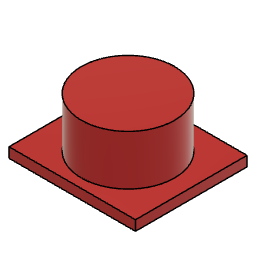
Buttons_V1 (Autodesk Fusion 360 archive; units mm, degrees)
design "ButtonRed"
Autodesk Fusion 360 part; units mm, degrees
(part 1 of 2)
sketch "Sketch1" plane through (0, 45, 0) normal (0, 1, 0) x (-1, 0, 0)
  line L0 (-111.8498, 7.1011) -> (-111.8498, -10.2989)
  line L1 (-111.8498, -10.2989) -> (-134.2498, -10.2989)
  line L2 (-134.2498, -10.2989) -> (-134.2498, 7.1011)
  line L3 (-134.2498, 7.1011) -> (-111.8498, 7.1011)
  circle A0 centre (-138.4498, -1.5989) radius 3.1
  circle A1 centre (-123.0498, 11.3011) radius 3.1
  circle A2 centre (-123.0498, -14.4989) radius 3.1
  circle A3 centre (-107.6498, -1.5989) radius 3.1
  line L4 (-103.4498, -18.6989) -> (-103.4498, 15.5011)
  line L5 (-103.4498, 15.5011) -> (-142.6498, 15.5011)
  line L6 (-142.6498, 15.5011) -> (-142.6498, -18.6989)
  line L7 (-142.6498, -18.6989) -> (-103.4498, -18.6989)
  circle A4 centre (-138.4498, -1.5989) radius 3.1
  circle A5 centre (-123.0498, -14.4989) radius 3.1
  circle A6 centre (-107.6498, -1.5989) radius 3.1
  circle A7 centre (-123.0498, 11.3011) radius 3.1
  line L8 (-154.8498, 7.1011) -> (-154.8498, -10.2989)
  line L9 (-177.2498, -10.2989) -> (-177.2498, 7.1011)
  line L10 (-146.7095, 15.4507) -> (-185.4095, 15.5014)
  line L11 (-177.2498, 7.1011) -> (-154.8498, 7.1011)
  circle A8 centre (-166.0498, -14.4989) radius 3.1
  circle A9 centre (-181.4498, -1.5989) radius 3.1
  line L12 (-185.4095, 15.5014) -> (-185.4536, -18.1986)
  circle A10 centre (-181.4498, -1.5989) radius 3.1
  line L13 (-146.7537, -18.2493) -> (-146.7095, 15.4507)
  circle A11 centre (-166.0498, 11.3011) radius 3.1
  circle A12 centre (-166.0498, 11.3011) radius 3.1
  line L14 (-154.8498, -10.2989) -> (-177.2498, -10.2989)
  circle A13 centre (-150.6498, -1.5989) radius 3.1
  circle A14 centre (-150.6498, -1.5989) radius 3.1
  line L15 (-185.4536, -18.1986) -> (-146.7537, -18.2493)
  circle A15 centre (-166.0498, -14.4989) radius 3.1
  arc A16 (86.5, -27.2432) -> (86.5, -22.3568) centre (88.5, -24.8) ccw
  arc A17 (-86.5, -22.3568) -> (-86.5, -27.2432) centre (-88.5, -24.8) ccw
  line L16 (86.5, 29) -> (-86.5, 29)
  line L17 (-86.5, 29) -> (-86.5, 27.2432)
  line L18 (-86.5, -29) -> (86.5, -29)
  line L19 (86.5, -29) -> (86.5, -27.2432)
  arc A18 (86.5, 22.3568) -> (86.5, 27.2432) centre (88.5, 24.8) ccw
  arc A19 (-86.5, 27.2432) -> (-86.5, 22.3568) centre (-88.5, 24.8) ccw
  line L20 (-86.5, 22.3568) -> (-86.5, -22.3568)
  line L21 (-86.5, -27.2432) -> (-86.5, -29)
  line L22 (86.5, -22.3568) -> (86.5, 22.3568)
  line L23 (86.5, 27.2432) -> (86.5, 29)
  dimension "d623" = 39.2
  dimension "d624" = 38.7
  dimension "d625" = 33.7
  dimension "d921" = 0
  dimension "d922" = 0
  dimension "d923" = 0
  dimension "d924" = 0
  constraint perpendicular L12 L15
  constraint parallel L10 L15
  constraint parallel L12 L13
  measures "d623" distance of L4.start L6.end
  measures "d624" distance of L13.start L12.end
  measures "d625" vertical distance of L10.end L12.end
extrude "Extrude1" [suppressed]
sketch "Sketch2" plane through (0, 45, 0) normal (0, 1, 0) x (-1, 0, 0)
  line L0 (-142.6498, -18.6989) -> (-103.4498, -18.6989)
  line L1 (-103.4498, -18.6989) -> (-103.4498, 15.5011)
  line L2 (-103.4498, 15.5011) -> (-142.6498, 15.5011)
  line L3 (-142.6498, 15.5011) -> (-142.6498, -18.6989)
extrude "Extrude2" [suppressed]
sketch "Sketch3" plane through (0, 49.8, 0) normal (0, 1, 0) x (-1, 0, 0)
  line L0 (-142.6498, 15.5011) -> (-142.6498, -18.6989)
  line L1 (-142.6498, -18.6989) -> (-103.4498, -18.6989)
  line L2 (-103.4498, -18.6989) -> (-103.4498, 15.5011)
  line L3 (-103.4498, 15.5011) -> (-142.6498, 15.5011)
  circle A0 centre (-123.0498, -1.5989) radius 14
  dimension "d616" = 28
  dimension "d617" = 17.1
  dimension "d618" = 34.2
  dimension "d619" = 39.2
  dimension "d620" = 19.6
  measures "d616" diameter of A0
  measures "d617" distance of L1 A0.centre
  measures "d618" distance of L1 L3
  measures "d619" distance of L0 L2
  measures "d620" distance of L2 A0.centre
extrude "Extrude3" [suppressed]
sketch "Sketch4" plane through (0, 49.8, 0) normal (0, 1, 0) x (-1, 0, 0)
  circle A0 centre (-123.0498, -1.5989) radius 14
  line L0 (-142.6498, 15.5011) -> (-142.6498, -18.6989)
  line L1 (-142.6498, -18.6989) -> (-103.4498, -18.6989)
  line L2 (-103.4498, -18.6989) -> (-103.4498, 15.5011)
  line L3 (-103.4498, 15.5011) -> (-142.6498, 15.5011)
  line L4 (-103.9498, 15.0011) -> (-142.1498, 15.0011)
  line L5 (-142.1498, 15.0011) -> (-142.1498, -18.1989)
  line L6 (-142.1498, -18.1989) -> (-103.9498, -18.1989)
  line L7 (-103.9498, -18.1989) -> (-103.9498, 15.0011)
  dimension "d627" = -0.5
extrude "Extrude4" [suppressed]
sketch "Sketch10" plane through (0, 37.0807, 0) normal (0, 1, 0) x (-1, 0, 0)
  circle A0 centre (80.75, -16) radius 2.1574
  circle A1 centre (80.75, 16.2) radius 2.1574
  circle A2 centre (-80.25, -16) radius 2.1574
  circle A3 centre (-80.25, 16.2) radius 2.1574
  line L0 (-81.25, -11) -> (-83.25, -11)
  line L1 (-83.25, -11) -> (-83.25, -19)
  line L2 (-83.25, -19) -> (-75.25, -19)
  line L3 (-75.25, -19) -> (-75.25, -17)
  line L4 (-75.25, -17) -> (-44.95, -17)
  line L5 (-44.95, -17) -> (-44.95, -19)
  line L6 (-44.95, -19) -> (-36.95, -19)
  line L7 (-36.95, -19) -> (-36.95, -17)
  line L8 (-36.95, -17) -> (-3.75, -17)
  line L9 (-3.75, -17) -> (-3.75, -19)
  line L10 (-3.75, -19) -> (4.25, -19)
  line L11 (4.25, -19) -> (4.25, -17)
  line L12 (4.25, -17) -> (37.45, -17)
  line L13 (37.45, -17) -> (37.45, -19)
  line L14 (37.45, -19) -> (45.45, -19)
  line L15 (45.45, -19) -> (45.45, -17)
  line L16 (45.45, -17) -> (75.75, -17)
  line L17 (75.75, -17) -> (75.75, -19)
  line L18 (75.75, -19) -> (83.75, -19)
  line L19 (83.75, -19) -> (83.75, -11)
  line L20 (83.75, -11) -> (81.75, -11)
  line L21 (81.75, -11) -> (81.75, 11.2)
  line L22 (81.75, 11.2) -> (83.75, 11.2)
  line L23 (83.75, 11.2) -> (83.75, 19.2)
  line L24 (83.75, 19.2) -> (75.75, 19.2)
  line L25 (75.75, 19.2) -> (75.75, 17.2)
  line L26 (75.75, 17.2) -> (45.45, 17.2)
  line L27 (45.45, 17.2) -> (45.45, 19.2)
  line L28 (45.45, 19.2) -> (37.45, 19.2)
  line L29 (37.45, 19.2) -> (37.45, 17.2)
  line L30 (37.45, 17.2) -> (4.25, 17.2)
  line L31 (4.25, 17.2) -> (4.25, 19.2)
  line L32 (4.25, 19.2) -> (-3.75, 19.2)
  line L33 (-3.75, 19.2) -> (-3.75, 17.2)
  line L34 (-3.75, 17.2) -> (-36.95, 17.2)
  line L35 (-36.95, 17.2) -> (-36.95, 19.2)
  line L36 (-36.95, 19.2) -> (-44.95, 19.2)
  line L37 (-44.95, 19.2) -> (-44.95, 17.2)
  line L38 (-44.95, 17.2) -> (-75.25, 17.2)
  line L39 (-75.25, 17.2) -> (-75.25, 19.2)
  line L40 (-75.25, 19.2) -> (-83.25, 19.2)
  line L41 (-83.25, 19.2) -> (-83.25, 11.2)
  line L42 (-83.25, 11.2) -> (-81.25, 11.2)
  line L43 (-81.25, 11.2) -> (-81.25, -11)
  line L44 (-0.75, -11) -> (-0.75, 11.2)
  line L45 (-0.75, 11.2) -> (1.25, 11.2)
  line L46 (1.25, 11.2) -> (1.25, -11)
  line L47 (1.25, -11) -> (-0.75, -11)
  line L48 (-41.95, -11) -> (-41.95, 11.2)
  line L49 (-41.95, 11.2) -> (-39.95, 11.2)
  line L50 (-39.95, 11.2) -> (-39.95, -11)
  line L51 (-39.95, -11) -> (-41.95, -11)
  circle A4 centre (-61.55, 13) radius 3.1
  circle A5 centre (-20.35, 13) radius 3.1
  circle A6 centre (36.25, 0.1) radius 3.1
  circle A7 centre (77.45, 0.1) radius 3.1
  circle A8 centre (62.05, -12.8) radius 3.1
  circle A9 centre (20.85, -12.8) radius 3.1
  circle A10 centre (-4.95, 0.1) radius 3.1
  circle A11 centre (-61.55, -12.8) radius 3.1
  circle A12 centre (-46.15, 0.1) radius 3.1
  circle A13 centre (-20.35, -12.8) radius 3.1
  circle A14 centre (20.85, 13) radius 3.1
  circle A15 centre (62.05, 13) radius 3.1
  circle A16 centre (46.65, 0.1) radius 3.1
  circle A17 centre (5.45, 0.1) radius 3.1
  circle A18 centre (-35.75, 0.1) radius 3.1
  circle A19 centre (-76.95, 0.1) radius 3.1
  line L52 (9.65, 8.8) -> (32.05, 8.8)
  line L53 (32.05, 8.8) -> (32.05, -8.6)
  line L54 (32.05, -8.6) -> (9.65, -8.6)
  line L55 (9.65, -8.6) -> (9.65, 8.8)
  line L56 (-31.55, 8.8) -> (-9.15, 8.8)
  line L57 (-9.15, 8.8) -> (-9.15, -8.6)
  line L58 (-9.15, -8.6) -> (-31.55, -8.6)
  line L59 (-31.55, -8.6) -> (-31.55, 8.8)
  line L60 (73.25, 8.8) -> (73.25, -8.6)
  line L61 (73.25, -8.6) -> (50.85, -8.6)
  line L62 (50.85, -8.6) -> (50.85, 8.8)
  line L63 (50.85, 8.8) -> (73.25, 8.8)
  line L64 (-72.75, 8.8) -> (-50.35, 8.8)
  line L65 (-50.35, 8.8) -> (-50.35, -8.6)
  line L66 (-50.35, -8.6) -> (-72.75, -8.6)
  line L67 (-72.75, -8.6) -> (-72.75, 8.8)
  line L68 (42.45, 11.2) -> (42.45, -11)
  line L69 (42.45, -11) -> (40.45, -11)
  line L70 (40.45, -11) -> (40.45, 11.2)
  line L71 (40.45, 11.2) -> (42.45, 11.2)
  circle A20 centre (62.05, 13) radius 3.1
  circle A21 centre (46.65, 0.1) radius 3.1
  circle A22 centre (62.05, -12.8) radius 3.1
  circle A23 centre (77.45, 0.1) radius 3.1
sketch "Sketch5" plane through (0, 24.0807, 0) normal (0, 1, 0) x (-1, 0, 0)
  circle A0 centre (80.5, -16.1) radius 2.1574
  circle A1 centre (80.5, 16.1) radius 2.1574
  circle A2 centre (-80.5, -16.1) radius 2.1574
  circle A3 centre (-80.5, 16.1) radius 2.1574
  line L0 (-81.5, -11.1) -> (-83.5, -11.1)
  line L1 (-83.5, -11.1) -> (-83.5, -19.1)
  line L2 (-83.5, -19.1) -> (-75.5, -19.1)
  line L3 (-75.5, -19.1) -> (-75.5, -17.1)
  line L4 (-75.5, -17.1) -> (-45.2, -17.1)
  line L5 (-45.2, -17.1) -> (-45.2, -19.1)
  line L6 (-45.2, -19.1) -> (-37.2, -19.1)
  line L7 (-37.2, -19.1) -> (-37.2, -17.1)
  line L8 (-37.2, -17.1) -> (-4, -17.1)
  line L9 (-4, -17.1) -> (-4, -19.1)
  line L10 (-4, -19.1) -> (4, -19.1)
  line L11 (4, -19.1) -> (4, -17.1)
  line L12 (4, -17.1) -> (37.2, -17.1)
  line L13 (37.2, -17.1) -> (37.2, -19.1)
  line L14 (37.2, -19.1) -> (45.2, -19.1)
  line L15 (45.2, -19.1) -> (45.2, -17.1)
  line L16 (45.2, -17.1) -> (75.5, -17.1)
  line L17 (75.5, -17.1) -> (75.5, -19.1)
  line L18 (75.5, -19.1) -> (83.5, -19.1)
  line L19 (83.5, -19.1) -> (83.5, -11.1)
  line L20 (83.5, -11.1) -> (81.5, -11.1)
  line L21 (81.5, -11.1) -> (81.5, 11.1)
  line L22 (81.5, 11.1) -> (83.5, 11.1)
  line L23 (83.5, 11.1) -> (83.5, 19.1)
  line L24 (83.5, 19.1) -> (75.5, 19.1)
  line L25 (75.5, 19.1) -> (75.5, 17.1)
  line L26 (75.5, 17.1) -> (45.2, 17.1)
  line L27 (45.2, 17.1) -> (45.2, 19.1)
  line L28 (45.2, 19.1) -> (37.2, 19.1)
  line L29 (37.2, 19.1) -> (37.2, 17.1)
  line L30 (37.2, 17.1) -> (4, 17.1)
  line L31 (4, 17.1) -> (4, 19.1)
  line L32 (4, 19.1) -> (-4, 19.1)
  line L33 (-4, 19.1) -> (-4, 17.1)
  line L34 (-4, 17.1) -> (-37.2, 17.1)
  line L35 (-37.2, 17.1) -> (-37.2, 19.1)
  line L36 (-37.2, 19.1) -> (-45.2, 19.1)
  line L37 (-45.2, 19.1) -> (-45.2, 17.1)
  line L38 (-45.2, 17.1) -> (-75.5, 17.1)
  line L39 (-75.5, 17.1) -> (-75.5, 19.1)
  line L40 (-75.5, 19.1) -> (-83.5, 19.1)
  line L41 (-83.5, 19.1) -> (-83.5, 11.1)
  line L42 (-83.5, 11.1) -> (-81.5, 11.1)
  line L43 (-81.5, 11.1) -> (-81.5, -11.1)
  line L44 (-1, -11.1) -> (-1, 11.1)
  line L45 (-1, 11.1) -> (1, 11.1)
  line L46 (1, 11.1) -> (1, -11.1)
  line L47 (1, -11.1) -> (-1, -11.1)
  line L48 (-42.2, -11.1) -> (-42.2, 11.1)
  line L49 (-42.2, 11.1) -> (-40.2, 11.1)
  line L50 (-40.2, 11.1) -> (-40.2, -11.1)
  line L51 (-40.2, -11.1) -> (-42.2, -11.1)
  circle A4 centre (-61.8, 12.9) radius 3.1
  circle A5 centre (-20.6, 12.9) radius 3.1
  circle A6 centre (36, 0) radius 3.1
  circle A7 centre (77.2, 0) radius 3.1
  circle A8 centre (61.8, -12.9) radius 3.1
  circle A9 centre (20.6, -12.9) radius 3.1
  circle A10 centre (-5.2, 0) radius 3.1
  circle A11 centre (-61.8, -12.9) radius 3.1
  circle A12 centre (-46.4, 0) radius 3.1
  circle A13 centre (-20.6, -12.9) radius 3.1
  circle A14 centre (20.6, 12.9) radius 3.1
  circle A15 centre (61.8, 12.9) radius 3.1
  circle A16 centre (46.4, 0) radius 3.1
  circle A17 centre (5.2, 0) radius 3.1
  circle A18 centre (-36, 0) radius 3.1
  circle A19 centre (-77.2, 0) radius 3.1
  line L52 (9.4, 8.7) -> (31.8, 8.7)
  line L53 (31.8, 8.7) -> (31.8, -8.7)
  line L54 (31.8, -8.7) -> (9.4, -8.7)
  line L55 (9.4, -8.7) -> (9.4, 8.7)
  line L56 (-31.8, 8.7) -> (-9.4, 8.7)
  line L57 (-9.4, 8.7) -> (-9.4, -8.7)
  line L58 (-9.4, -8.7) -> (-31.8, -8.7)
  line L59 (-31.8, -8.7) -> (-31.8, 8.7)
  line L60 (73, 8.7) -> (73, -8.7)
  line L61 (73, -8.7) -> (50.6, -8.7)
  line L62 (50.6, -8.7) -> (50.6, 8.7)
  line L63 (50.6, 8.7) -> (73, 8.7)
  line L64 (-73, 8.7) -> (-50.6, 8.7)
  line L65 (-50.6, 8.7) -> (-50.6, -8.7)
  line L66 (-50.6, -8.7) -> (-73, -8.7)
  line L67 (-73, -8.7) -> (-73, 8.7)
  line L68 (42.2, 11.1) -> (42.2, -11.1)
  line L69 (42.2, -11.1) -> (40.2, -11.1)
  line L70 (40.2, -11.1) -> (40.2, 11.1)
  line L71 (40.2, 11.1) -> (42.2, 11.1)
  circle A20 centre (20.6, 12.9) radius 3.1
  line L72 (-1, -11.1) -> (1, -11.1)
  line L73 (1, -11.1) -> (1, 11.1)
  line L74 (1, 11.1) -> (-1, 11.1)
  line L75 (-1, 11.1) -> (-1, -11.1)
  circle A21 centre (20.6, -12.9) radius 3.1
  line L76 (4, -19.1) -> (37.2, -19.1)
  line L77 (37.2, -19.1) -> (37.2, -17.1)
  line L78 (37.2, -17.1) -> (4, -17.1)
  line L79 (4, -17.1) -> (4, -19.1)
  line L80 (42.2, 11.1) -> (40.2, 11.1)
  line L81 (40.2, 11.1) -> (40.2, -11.1)
  line L82 (40.2, -11.1) -> (42.2, -11.1)
  line L83 (42.2, -11.1) -> (42.2, 11.1)
  line L84 (37.2, 19.1) -> (4, 19.1)
  line L85 (4, 19.1) -> (4, 17.1)
  line L86 (4, 17.1) -> (37.2, 17.1)
  line L87 (37.2, 17.1) -> (37.2, 19.1)
  line L88 (39.6, -16.8333) -> (1.6, -16.8333)
  line L89 (1.6, -16.8333) -> (1.6, 16.6667)
  line L90 (1.6, 16.6667) -> (39.6, 16.6667)
  line L91 (39.6, 16.6667) -> (39.6, -16.8333)
  line L92 (39.6, -16.8333) -> (1.6, 16.6667) construction
  line L93 (1.6, -16.8333) -> (39.6, 16.6667) construction
  point P0 (5.2, 0)
  point P1 (20.6, -12.9)
  point P2 (20.6, -0.0833)
  dimension "d849" = 38
  dimension "d850" = 33.5
  dimension "d933" = 0
  dimension "d934" = 0
  dimension "d935" = 0
  constraint perpendicular L88 L89
  constraint parallel L88 L90
  constraint parallel L89 L91
  constraint horizontal L88
  constraint coincident L92 P2
  constraint coincident L93 P2
  measures "d849" distance of L89.end L90.end
  measures "d850" distance of L88.end L89.end
extrude "Extrude5" add sketch "Sketch5" against normal blind 1.8 contours L52 L53 L54 L55 | L88 L89 L90 L91
sketch "Sketch7" plane through (0, 24.0807, 0) normal (0, 1, 0) x (-1, 0, 0)
  circle A0 centre (20.6, -12.9) radius 3.1
  circle A1 centre (20.6, 12.9) radius 3.1
  circle A2 centre (5.2, 0) radius 3.1
  circle A3 centre (36, 0) radius 3.1
  line L0 (39.6, 16.6667) -> (1.6, 16.6667)
  line L1 (1.6, 16.6667) -> (1.6, -16.8333)
  line L2 (1.6, -16.8333) -> (39.6, -16.8333)
  line L3 (39.6, -16.8333) -> (39.6, 16.6667)
  line L4 (39.6, -16.8333) -> (1.6, -16.8333)
  line L5 (1.6, -16.8333) -> (1.6, 16.6667)
  line L6 (1.6, 16.6667) -> (39.6, 16.6667)
  line L7 (39.6, 16.6667) -> (39.6, -16.8333)
  dimension "d859" = 38
  constraint horizontal L4
  constraint vertical L5
  constraint horizontal L6
  constraint vertical L7
  constraint coincident L0.end L1.start
  constraint coincident L2.end L3.start
  measures "d859" distance of L2.end L1.end
extrude "Extrude7" add sketch "Sketch7" along normal blind 1.2 contours A0 | A1 | A2 | A3 | L0 L1 L2 L3 L4 L5 L6 L7
sketch "Sketch8" plane through (0, 25.2807, 0) normal (0, 1, 0) x (-1, 0, 0)
  line L0 (39.6, 16.6667) -> (1.6, 16.6667)
  line L1 (1.6, 16.6667) -> (1.6, -16.8333)
  line L2 (1.6, -16.8333) -> (39.6, -16.8333)
  line L3 (39.6, -16.8333) -> (39.6, 16.6667)
  circle A0 centre (20.6, -0.0833) radius 14
  dimension "d862" = 19
  dimension "d863" = 16.75
  dimension "d864" = 28
  dimension "d865" = 38
  dimension "d866" = 33.5
  measures "d862" distance of L1 A0.centre
  measures "d863" distance of L0 A0.centre
  measures "d864" diameter of A0
  measures "d865" distance of L1.end L2.end
  measures "d866" distance of L0.start L2.end
extrude "Extrude8" add sketch "Sketch8" along normal blind 15 contours A0
sketch "Sketch9" plane through (-1.6, 0, 0) normal (1, 0, 0) x (0, 0, -1)
  line L0 (-16.6667, 25.2807) -> (-16.6667, 22.2807)
  line L1 (-16.6667, 22.2807) -> (16.8333, 22.2807)
  line L2 (16.8333, 22.2807) -> (16.8333, 25.2807)
  line L3 (16.8333, 25.2807) -> (-16.6667, 25.2807)
component "Component" placed x (1, 0, 0) y (0, 1, 0) z (0, 0, 1) at (0, 0, 0)
equation "d612 = magnetDepth"
equation "d614 = 3 mm - magnetDepth"
equation "d616 = buttonOD"
equation "d617 = ( 34.2 / 2 ) * 1 mm"
equation "d620 = ( 39.2 / 2 ) * 1 mm"
equation "d621 = buttonH"
equation "d624 = 39.2 mm - 0.5 mm"
equation "d625 = 34.2 mm - 0.5 mm"
equation "d850 = buttonBaseW"
equation "d853 = magnetDepth"
equation "d860 = 3 mm + magnetDepth"
equation "d862 = ( 38 / 2 ) * 1 mm"
equation "d863 = ( 33.5 / 2 ) * 1 mm"
equation "d864 = buttonOD"
equation "d867 = buttonH"
equation "buttonOD = 28 mm"
equation "buttonH = 15 mm"
equation "magnetDepth = -1.8 mm" comment "1.43 mm"
equation "buttonBaseW = 33.5 mm"

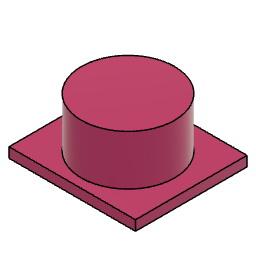
design "ButtonPink"
Autodesk Fusion 360 part; units mm, degrees
sketch "Sketch1" plane through (0, 45, 0) normal (0, 1, 0) x (-1, 0, 0)
  line L0 (-111.8498, 7.1011) -> (-111.8498, -10.2989)
  line L1 (-111.8498, -10.2989) -> (-134.2498, -10.2989)
  line L2 (-134.2498, -10.2989) -> (-134.2498, 7.1011)
  line L3 (-134.2498, 7.1011) -> (-111.8498, 7.1011)
  circle A0 centre (-138.4498, -1.5989) radius 3.1
  circle A1 centre (-123.0498, 11.3011) radius 3.1
  circle A2 centre (-123.0498, -14.4989) radius 3.1
  circle A3 centre (-107.6498, -1.5989) radius 3.1
  line L4 (-103.4498, -18.6989) -> (-103.4498, 15.5011)
  line L5 (-103.4498, 15.5011) -> (-142.6498, 15.5011)
  line L6 (-142.6498, 15.5011) -> (-142.6498, -18.6989)
  line L7 (-142.6498, -18.6989) -> (-103.4498, -18.6989)
  circle A4 centre (-138.4498, -1.5989) radius 3.1
  circle A5 centre (-123.0498, -14.4989) radius 3.1
  circle A6 centre (-107.6498, -1.5989) radius 3.1
  circle A7 centre (-123.0498, 11.3011) radius 3.1
  line L8 (-154.8498, 7.1011) -> (-154.8498, -10.2989)
  line L9 (-177.2498, -10.2989) -> (-177.2498, 7.1011)
  line L10 (-146.7095, 15.4507) -> (-185.4095, 15.5014)
  line L11 (-177.2498, 7.1011) -> (-154.8498, 7.1011)
  circle A8 centre (-166.0498, -14.4989) radius 3.1
  circle A9 centre (-181.4498, -1.5989) radius 3.1
  line L12 (-185.4095, 15.5014) -> (-185.4536, -18.1986)
  circle A10 centre (-181.4498, -1.5989) radius 3.1
  line L13 (-146.7537, -18.2493) -> (-146.7095, 15.4507)
  circle A11 centre (-166.0498, 11.3011) radius 3.1
  circle A12 centre (-166.0498, 11.3011) radius 3.1
  line L14 (-154.8498, -10.2989) -> (-177.2498, -10.2989)
  circle A13 centre (-150.6498, -1.5989) radius 3.1
  circle A14 centre (-150.6498, -1.5989) radius 3.1
  line L15 (-185.4536, -18.1986) -> (-146.7537, -18.2493)
  circle A15 centre (-166.0498, -14.4989) radius 3.1
  arc A16 (86.5, -27.2432) -> (86.5, -22.3568) centre (88.5, -24.8) ccw
  arc A17 (-86.5, -22.3568) -> (-86.5, -27.2432) centre (-88.5, -24.8) ccw
  line L16 (86.5, 29) -> (-86.5, 29)
  line L17 (-86.5, 29) -> (-86.5, 27.2432)
  line L18 (-86.5, -29) -> (86.5, -29)
  line L19 (86.5, -29) -> (86.5, -27.2432)
  arc A18 (86.5, 22.3568) -> (86.5, 27.2432) centre (88.5, 24.8) ccw
  arc A19 (-86.5, 27.2432) -> (-86.5, 22.3568) centre (-88.5, 24.8) ccw
  line L20 (-86.5, 22.3568) -> (-86.5, -22.3568)
  line L21 (-86.5, -27.2432) -> (-86.5, -29)
  line L22 (86.5, -22.3568) -> (86.5, 22.3568)
  line L23 (86.5, 27.2432) -> (86.5, 29)
  dimension "d623" = 39.2
  dimension "d624" = 38.7
  dimension "d625" = 33.7
  dimension "d921" = 0
  dimension "d922" = 0
  dimension "d923" = 0
  dimension "d924" = 0
  constraint perpendicular L12 L15
  constraint parallel L10 L15
  constraint parallel L12 L13
  measures "d623" distance of L4.start L6.end
  measures "d624" distance of L13.start L12.end
  measures "d625" vertical distance of L10.end L12.end
extrude "Extrude1" [suppressed]
sketch "Sketch2" plane through (0, 45, 0) normal (0, 1, 0) x (-1, 0, 0)
  line L0 (-142.6498, -18.6989) -> (-103.4498, -18.6989)
  line L1 (-103.4498, -18.6989) -> (-103.4498, 15.5011)
  line L2 (-103.4498, 15.5011) -> (-142.6498, 15.5011)
  line L3 (-142.6498, 15.5011) -> (-142.6498, -18.6989)
extrude "Extrude2" [suppressed]
sketch "Sketch3" plane through (0, 49.8, 0) normal (0, 1, 0) x (-1, 0, 0)
  line L0 (-142.6498, 15.5011) -> (-142.6498, -18.6989)
  line L1 (-142.6498, -18.6989) -> (-103.4498, -18.6989)
  line L2 (-103.4498, -18.6989) -> (-103.4498, 15.5011)
  line L3 (-103.4498, 15.5011) -> (-142.6498, 15.5011)
  circle A0 centre (-123.0498, -1.5989) radius 14
  dimension "d616" = 28
  dimension "d617" = 17.1
  dimension "d618" = 34.2
  dimension "d619" = 39.2
  dimension "d620" = 19.6
  measures "d616" diameter of A0
  measures "d617" distance of L1 A0.centre
  measures "d618" distance of L1 L3
  measures "d619" distance of L0 L2
  measures "d620" distance of L2 A0.centre
extrude "Extrude3" [suppressed]
sketch "Sketch4" plane through (0, 49.8, 0) normal (0, 1, 0) x (-1, 0, 0)
  circle A0 centre (-123.0498, -1.5989) radius 14
  line L0 (-142.6498, 15.5011) -> (-142.6498, -18.6989)
  line L1 (-142.6498, -18.6989) -> (-103.4498, -18.6989)
  line L2 (-103.4498, -18.6989) -> (-103.4498, 15.5011)
  line L3 (-103.4498, 15.5011) -> (-142.6498, 15.5011)
  line L4 (-103.9498, 15.0011) -> (-142.1498, 15.0011)
  line L5 (-142.1498, 15.0011) -> (-142.1498, -18.1989)
  line L6 (-142.1498, -18.1989) -> (-103.9498, -18.1989)
  line L7 (-103.9498, -18.1989) -> (-103.9498, 15.0011)
  dimension "d627" = -0.5
extrude "Extrude4" [suppressed]
sketch "Sketch10" plane through (0, 37.0807, 0) normal (0, 1, 0) x (-1, 0, 0)
  circle A0 centre (80.75, -16) radius 2.1574
  circle A1 centre (80.75, 16.2) radius 2.1574
  circle A2 centre (-80.25, -16) radius 2.1574
  circle A3 centre (-80.25, 16.2) radius 2.1574
  line L0 (-81.25, -11) -> (-83.25, -11)
  line L1 (-83.25, -11) -> (-83.25, -19)
  line L2 (-83.25, -19) -> (-75.25, -19)
  line L3 (-75.25, -19) -> (-75.25, -17)
  line L4 (-75.25, -17) -> (-44.95, -17)
  line L5 (-44.95, -17) -> (-44.95, -19)
  line L6 (-44.95, -19) -> (-36.95, -19)
  line L7 (-36.95, -19) -> (-36.95, -17)
  line L8 (-36.95, -17) -> (-3.75, -17)
  line L9 (-3.75, -17) -> (-3.75, -19)
  line L10 (-3.75, -19) -> (4.25, -19)
  line L11 (4.25, -19) -> (4.25, -17)
  line L12 (4.25, -17) -> (37.45, -17)
  line L13 (37.45, -17) -> (37.45, -19)
  line L14 (37.45, -19) -> (45.45, -19)
  line L15 (45.45, -19) -> (45.45, -17)
  line L16 (45.45, -17) -> (75.75, -17)
  line L17 (75.75, -17) -> (75.75, -19)
  line L18 (75.75, -19) -> (83.75, -19)
  line L19 (83.75, -19) -> (83.75, -11)
  line L20 (83.75, -11) -> (81.75, -11)
  line L21 (81.75, -11) -> (81.75, 11.2)
  line L22 (81.75, 11.2) -> (83.75, 11.2)
  line L23 (83.75, 11.2) -> (83.75, 19.2)
  line L24 (83.75, 19.2) -> (75.75, 19.2)
  line L25 (75.75, 19.2) -> (75.75, 17.2)
  line L26 (75.75, 17.2) -> (45.45, 17.2)
  line L27 (45.45, 17.2) -> (45.45, 19.2)
  line L28 (45.45, 19.2) -> (37.45, 19.2)
  line L29 (37.45, 19.2) -> (37.45, 17.2)
  line L30 (37.45, 17.2) -> (4.25, 17.2)
  line L31 (4.25, 17.2) -> (4.25, 19.2)
  line L32 (4.25, 19.2) -> (-3.75, 19.2)
  line L33 (-3.75, 19.2) -> (-3.75, 17.2)
  line L34 (-3.75, 17.2) -> (-36.95, 17.2)
  line L35 (-36.95, 17.2) -> (-36.95, 19.2)
  line L36 (-36.95, 19.2) -> (-44.95, 19.2)
  line L37 (-44.95, 19.2) -> (-44.95, 17.2)
  line L38 (-44.95, 17.2) -> (-75.25, 17.2)
  line L39 (-75.25, 17.2) -> (-75.25, 19.2)
  line L40 (-75.25, 19.2) -> (-83.25, 19.2)
  line L41 (-83.25, 19.2) -> (-83.25, 11.2)
  line L42 (-83.25, 11.2) -> (-81.25, 11.2)
  line L43 (-81.25, 11.2) -> (-81.25, -11)
  line L44 (-0.75, -11) -> (-0.75, 11.2)
  line L45 (-0.75, 11.2) -> (1.25, 11.2)
  line L46 (1.25, 11.2) -> (1.25, -11)
  line L47 (1.25, -11) -> (-0.75, -11)
  line L48 (-41.95, -11) -> (-41.95, 11.2)
  line L49 (-41.95, 11.2) -> (-39.95, 11.2)
  line L50 (-39.95, 11.2) -> (-39.95, -11)
  line L51 (-39.95, -11) -> (-41.95, -11)
  circle A4 centre (-61.55, 13) radius 3.1
  circle A5 centre (-20.35, 13) radius 3.1
  circle A6 centre (36.25, 0.1) radius 3.1
  circle A7 centre (77.45, 0.1) radius 3.1
  circle A8 centre (62.05, -12.8) radius 3.1
  circle A9 centre (20.85, -12.8) radius 3.1
  circle A10 centre (-4.95, 0.1) radius 3.1
  circle A11 centre (-61.55, -12.8) radius 3.1
  circle A12 centre (-46.15, 0.1) radius 3.1
  circle A13 centre (-20.35, -12.8) radius 3.1
  circle A14 centre (20.85, 13) radius 3.1
  circle A15 centre (62.05, 13) radius 3.1
  circle A16 centre (46.65, 0.1) radius 3.1
  circle A17 centre (5.45, 0.1) radius 3.1
  circle A18 centre (-35.75, 0.1) radius 3.1
  circle A19 centre (-76.95, 0.1) radius 3.1
  line L52 (9.65, 8.8) -> (32.05, 8.8)
  line L53 (32.05, 8.8) -> (32.05, -8.6)
  line L54 (32.05, -8.6) -> (9.65, -8.6)
  line L55 (9.65, -8.6) -> (9.65, 8.8)
  line L56 (-31.55, 8.8) -> (-9.15, 8.8)
  line L57 (-9.15, 8.8) -> (-9.15, -8.6)
  line L58 (-9.15, -8.6) -> (-31.55, -8.6)
  line L59 (-31.55, -8.6) -> (-31.55, 8.8)
  line L60 (73.25, 8.8) -> (73.25, -8.6)
  line L61 (73.25, -8.6) -> (50.85, -8.6)
  line L62 (50.85, -8.6) -> (50.85, 8.8)
  line L63 (50.85, 8.8) -> (73.25, 8.8)
  line L64 (-72.75, 8.8) -> (-50.35, 8.8)
  line L65 (-50.35, 8.8) -> (-50.35, -8.6)
  line L66 (-50.35, -8.6) -> (-72.75, -8.6)
  line L67 (-72.75, -8.6) -> (-72.75, 8.8)
  line L68 (42.45, 11.2) -> (42.45, -11)
  line L69 (42.45, -11) -> (40.45, -11)
  line L70 (40.45, -11) -> (40.45, 11.2)
  line L71 (40.45, 11.2) -> (42.45, 11.2)
  circle A20 centre (62.05, 13) radius 3.1
  circle A21 centre (46.65, 0.1) radius 3.1
  circle A22 centre (62.05, -12.8) radius 3.1
  circle A23 centre (77.45, 0.1) radius 3.1
sketch "Sketch5" plane through (0, 24.0807, 0) normal (0, 1, 0) x (-1, 0, 0)
  circle A0 centre (80.5, -16.1) radius 2.1574
  circle A1 centre (80.5, 16.1) radius 2.1574
  circle A2 centre (-80.5, -16.1) radius 2.1574
  circle A3 centre (-80.5, 16.1) radius 2.1574
  line L0 (-81.5, -11.1) -> (-83.5, -11.1)
  line L1 (-83.5, -11.1) -> (-83.5, -19.1)
  line L2 (-83.5, -19.1) -> (-75.5, -19.1)
  line L3 (-75.5, -19.1) -> (-75.5, -17.1)
  line L4 (-75.5, -17.1) -> (-45.2, -17.1)
  line L5 (-45.2, -17.1) -> (-45.2, -19.1)
  line L6 (-45.2, -19.1) -> (-37.2, -19.1)
  line L7 (-37.2, -19.1) -> (-37.2, -17.1)
  line L8 (-37.2, -17.1) -> (-4, -17.1)
  line L9 (-4, -17.1) -> (-4, -19.1)
  line L10 (-4, -19.1) -> (4, -19.1)
  line L11 (4, -19.1) -> (4, -17.1)
  line L12 (4, -17.1) -> (37.2, -17.1)
  line L13 (37.2, -17.1) -> (37.2, -19.1)
  line L14 (37.2, -19.1) -> (45.2, -19.1)
  line L15 (45.2, -19.1) -> (45.2, -17.1)
  line L16 (45.2, -17.1) -> (75.5, -17.1)
  line L17 (75.5, -17.1) -> (75.5, -19.1)
  line L18 (75.5, -19.1) -> (83.5, -19.1)
  line L19 (83.5, -19.1) -> (83.5, -11.1)
  line L20 (83.5, -11.1) -> (81.5, -11.1)
  line L21 (81.5, -11.1) -> (81.5, 11.1)
  line L22 (81.5, 11.1) -> (83.5, 11.1)
  line L23 (83.5, 11.1) -> (83.5, 19.1)
  line L24 (83.5, 19.1) -> (75.5, 19.1)
  line L25 (75.5, 19.1) -> (75.5, 17.1)
  line L26 (75.5, 17.1) -> (45.2, 17.1)
  line L27 (45.2, 17.1) -> (45.2, 19.1)
  line L28 (45.2, 19.1) -> (37.2, 19.1)
  line L29 (37.2, 19.1) -> (37.2, 17.1)
  line L30 (37.2, 17.1) -> (4, 17.1)
  line L31 (4, 17.1) -> (4, 19.1)
  line L32 (4, 19.1) -> (-4, 19.1)
  line L33 (-4, 19.1) -> (-4, 17.1)
  line L34 (-4, 17.1) -> (-37.2, 17.1)
  line L35 (-37.2, 17.1) -> (-37.2, 19.1)
  line L36 (-37.2, 19.1) -> (-45.2, 19.1)
  line L37 (-45.2, 19.1) -> (-45.2, 17.1)
  line L38 (-45.2, 17.1) -> (-75.5, 17.1)
  line L39 (-75.5, 17.1) -> (-75.5, 19.1)
  line L40 (-75.5, 19.1) -> (-83.5, 19.1)
  line L41 (-83.5, 19.1) -> (-83.5, 11.1)
  line L42 (-83.5, 11.1) -> (-81.5, 11.1)
  line L43 (-81.5, 11.1) -> (-81.5, -11.1)
  line L44 (-1, -11.1) -> (-1, 11.1)
  line L45 (-1, 11.1) -> (1, 11.1)
  line L46 (1, 11.1) -> (1, -11.1)
  line L47 (1, -11.1) -> (-1, -11.1)
  line L48 (-42.2, -11.1) -> (-42.2, 11.1)
  line L49 (-42.2, 11.1) -> (-40.2, 11.1)
  line L50 (-40.2, 11.1) -> (-40.2, -11.1)
  line L51 (-40.2, -11.1) -> (-42.2, -11.1)
  circle A4 centre (-61.8, 12.9) radius 3.1
  circle A5 centre (-20.6, 12.9) radius 3.1
  circle A6 centre (36, 0) radius 3.1
  circle A7 centre (77.2, 0) radius 3.1
  circle A8 centre (61.8, -12.9) radius 3.1
  circle A9 centre (20.6, -12.9) radius 3.1
  circle A10 centre (-5.2, 0) radius 3.1
  circle A11 centre (-61.8, -12.9) radius 3.1
  circle A12 centre (-46.4, 0) radius 3.1
  circle A13 centre (-20.6, -12.9) radius 3.1
  circle A14 centre (20.6, 12.9) radius 3.1
  circle A15 centre (61.8, 12.9) radius 3.1
  circle A16 centre (46.4, 0) radius 3.1
  circle A17 centre (5.2, 0) radius 3.1
  circle A18 centre (-36, 0) radius 3.1
  circle A19 centre (-77.2, 0) radius 3.1
  line L52 (9.4, 8.7) -> (31.8, 8.7)
  line L53 (31.8, 8.7) -> (31.8, -8.7)
  line L54 (31.8, -8.7) -> (9.4, -8.7)
  line L55 (9.4, -8.7) -> (9.4, 8.7)
  line L56 (-31.8, 8.7) -> (-9.4, 8.7)
  line L57 (-9.4, 8.7) -> (-9.4, -8.7)
  line L58 (-9.4, -8.7) -> (-31.8, -8.7)
  line L59 (-31.8, -8.7) -> (-31.8, 8.7)
  line L60 (73, 8.7) -> (73, -8.7)
  line L61 (73, -8.7) -> (50.6, -8.7)
  line L62 (50.6, -8.7) -> (50.6, 8.7)
  line L63 (50.6, 8.7) -> (73, 8.7)
  line L64 (-73, 8.7) -> (-50.6, 8.7)
  line L65 (-50.6, 8.7) -> (-50.6, -8.7)
  line L66 (-50.6, -8.7) -> (-73, -8.7)
  line L67 (-73, -8.7) -> (-73, 8.7)
  line L68 (42.2, 11.1) -> (42.2, -11.1)
  line L69 (42.2, -11.1) -> (40.2, -11.1)
  line L70 (40.2, -11.1) -> (40.2, 11.1)
  line L71 (40.2, 11.1) -> (42.2, 11.1)
  circle A20 centre (20.6, 12.9) radius 3.1
  line L72 (-1, -11.1) -> (1, -11.1)
  line L73 (1, -11.1) -> (1, 11.1)
  line L74 (1, 11.1) -> (-1, 11.1)
  line L75 (-1, 11.1) -> (-1, -11.1)
  circle A21 centre (20.6, -12.9) radius 3.1
  line L76 (4, -19.1) -> (37.2, -19.1)
  line L77 (37.2, -19.1) -> (37.2, -17.1)
  line L78 (37.2, -17.1) -> (4, -17.1)
  line L79 (4, -17.1) -> (4, -19.1)
  line L80 (42.2, 11.1) -> (40.2, 11.1)
  line L81 (40.2, 11.1) -> (40.2, -11.1)
  line L82 (40.2, -11.1) -> (42.2, -11.1)
  line L83 (42.2, -11.1) -> (42.2, 11.1)
  line L84 (37.2, 19.1) -> (4, 19.1)
  line L85 (4, 19.1) -> (4, 17.1)
  line L86 (4, 17.1) -> (37.2, 17.1)
  line L87 (37.2, 17.1) -> (37.2, 19.1)
  line L88 (39.6, -16.8333) -> (1.6, -16.8333)
  line L89 (1.6, -16.8333) -> (1.6, 16.6667)
  line L90 (1.6, 16.6667) -> (39.6, 16.6667)
  line L91 (39.6, 16.6667) -> (39.6, -16.8333)
  line L92 (39.6, -16.8333) -> (1.6, 16.6667) construction
  line L93 (1.6, -16.8333) -> (39.6, 16.6667) construction
  point P0 (5.2, 0)
  point P1 (20.6, -12.9)
  point P2 (20.6, -0.0833)
  dimension "d849" = 38
  dimension "d850" = 33.5
  dimension "d933" = 0
  dimension "d934" = 0
  dimension "d935" = 0
  constraint perpendicular L88 L89
  constraint parallel L88 L90
  constraint parallel L89 L91
  constraint horizontal L88
  constraint coincident L92 P2
  constraint coincident L93 P2
  measures "d849" distance of L89.end L90.end
  measures "d850" distance of L88.end L89.end
extrude "Extrude5" add sketch "Sketch5" against normal blind 1.8 contours L52 L53 L54 L55 | L88 L89 L90 L91
sketch "Sketch7" plane through (0, 24.0807, 0) normal (0, 1, 0) x (-1, 0, 0)
  circle A0 centre (20.6, -12.9) radius 3.1
  circle A1 centre (20.6, 12.9) radius 3.1
  circle A2 centre (5.2, 0) radius 3.1
  circle A3 centre (36, 0) radius 3.1
  line L0 (39.6, 16.6667) -> (1.6, 16.6667)
  line L1 (1.6, 16.6667) -> (1.6, -16.8333)
  line L2 (1.6, -16.8333) -> (39.6, -16.8333)
  line L3 (39.6, -16.8333) -> (39.6, 16.6667)
  line L4 (39.6, -16.8333) -> (1.6, -16.8333)
  line L5 (1.6, -16.8333) -> (1.6, 16.6667)
  line L6 (1.6, 16.6667) -> (39.6, 16.6667)
  line L7 (39.6, 16.6667) -> (39.6, -16.8333)
  dimension "d859" = 38
  constraint horizontal L4
  constraint vertical L5
  constraint horizontal L6
  constraint vertical L7
  constraint coincident L0.end L1.start
  constraint coincident L2.end L3.start
  measures "d859" distance of L2.end L1.end
extrude "Extrude7" add sketch "Sketch7" along normal blind 1.2 contours A0 | A1 | A2 | A3 | L0 L1 L2 L3 L4 L5 L6 L7
sketch "Sketch8" plane through (0, 25.2807, 0) normal (0, 1, 0) x (-1, 0, 0)
  line L0 (39.6, 16.6667) -> (1.6, 16.6667)
  line L1 (1.6, 16.6667) -> (1.6, -16.8333)
  line L2 (1.6, -16.8333) -> (39.6, -16.8333)
  line L3 (39.6, -16.8333) -> (39.6, 16.6667)
  circle A0 centre (20.6, -0.0833) radius 14
  dimension "d862" = 19
  dimension "d863" = 16.75
  dimension "d864" = 28
  dimension "d865" = 38
  dimension "d866" = 33.5
  measures "d862" distance of L1 A0.centre
  measures "d863" distance of L0 A0.centre
  measures "d864" diameter of A0
  measures "d865" distance of L1.end L2.end
  measures "d866" distance of L0.start L2.end
extrude "Extrude8" add sketch "Sketch8" along normal blind 15 contours A0
sketch "Sketch9" plane through (-1.6, 0, 0) normal (1, 0, 0) x (0, 0, -1)
  line L0 (-16.6667, 25.2807) -> (-16.6667, 22.2807)
  line L1 (-16.6667, 22.2807) -> (16.8333, 22.2807)
  line L2 (16.8333, 22.2807) -> (16.8333, 25.2807)
  line L3 (16.8333, 25.2807) -> (-16.6667, 25.2807)
component "Component" placed x (1, 0, 0) y (0, 1, 0) z (0, 0, 1) at (0, 0, 0)
equation "d612 = magnetDepth"
equation "d614 = 3 mm - magnetDepth"
equation "d616 = buttonOD"
equation "d617 = ( 34.2 / 2 ) * 1 mm"
equation "d620 = ( 39.2 / 2 ) * 1 mm"
equation "d621 = buttonH"
equation "d624 = 39.2 mm - 0.5 mm"
equation "d625 = 34.2 mm - 0.5 mm"
equation "d850 = buttonBaseW"
equation "d853 = magnetDepth"
equation "d860 = 3 mm + magnetDepth"
equation "d862 = ( 38 / 2 ) * 1 mm"
equation "d863 = ( 33.5 / 2 ) * 1 mm"
equation "d864 = buttonOD"
equation "d867 = buttonH"
equation "buttonOD = 28 mm"
equation "buttonH = 15 mm"
equation "magnetDepth = -1.8 mm" comment "1.43 mm"
equation "buttonBaseW = 33.5 mm"

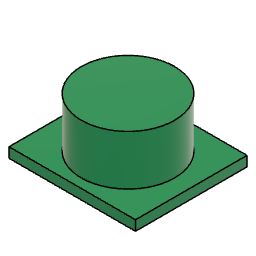
design "ButtonGreen"
Autodesk Fusion 360 part; units mm, degrees
sketch "Sketch1" plane through (0, 45, 0) normal (0, 1, 0) x (-1, 0, 0)
  line L0 (-111.8498, 7.1011) -> (-111.8498, -10.2989)
  line L1 (-111.8498, -10.2989) -> (-134.2498, -10.2989)
  line L2 (-134.2498, -10.2989) -> (-134.2498, 7.1011)
  line L3 (-134.2498, 7.1011) -> (-111.8498, 7.1011)
  circle A0 centre (-138.4498, -1.5989) radius 3.1
  circle A1 centre (-123.0498, 11.3011) radius 3.1
  circle A2 centre (-123.0498, -14.4989) radius 3.1
  circle A3 centre (-107.6498, -1.5989) radius 3.1
  line L4 (-103.4498, -18.6989) -> (-103.4498, 15.5011)
  line L5 (-103.4498, 15.5011) -> (-142.6498, 15.5011)
  line L6 (-142.6498, 15.5011) -> (-142.6498, -18.6989)
  line L7 (-142.6498, -18.6989) -> (-103.4498, -18.6989)
  circle A4 centre (-138.4498, -1.5989) radius 3.1
  circle A5 centre (-123.0498, -14.4989) radius 3.1
  circle A6 centre (-107.6498, -1.5989) radius 3.1
  circle A7 centre (-123.0498, 11.3011) radius 3.1
  line L8 (-154.8498, 7.1011) -> (-154.8498, -10.2989)
  line L9 (-177.2498, -10.2989) -> (-177.2498, 7.1011)
  line L10 (-146.7095, 15.4507) -> (-185.4095, 15.5014)
  line L11 (-177.2498, 7.1011) -> (-154.8498, 7.1011)
  circle A8 centre (-166.0498, -14.4989) radius 3.1
  circle A9 centre (-181.4498, -1.5989) radius 3.1
  line L12 (-185.4095, 15.5014) -> (-185.4536, -18.1986)
  circle A10 centre (-181.4498, -1.5989) radius 3.1
  line L13 (-146.7537, -18.2493) -> (-146.7095, 15.4507)
  circle A11 centre (-166.0498, 11.3011) radius 3.1
  circle A12 centre (-166.0498, 11.3011) radius 3.1
  line L14 (-154.8498, -10.2989) -> (-177.2498, -10.2989)
  circle A13 centre (-150.6498, -1.5989) radius 3.1
  circle A14 centre (-150.6498, -1.5989) radius 3.1
  line L15 (-185.4536, -18.1986) -> (-146.7537, -18.2493)
  circle A15 centre (-166.0498, -14.4989) radius 3.1
  arc A16 (86.5, -27.2432) -> (86.5, -22.3568) centre (88.5, -24.8) ccw
  arc A17 (-86.5, -22.3568) -> (-86.5, -27.2432) centre (-88.5, -24.8) ccw
  line L16 (86.5, 29) -> (-86.5, 29)
  line L17 (-86.5, 29) -> (-86.5, 27.2432)
  line L18 (-86.5, -29) -> (86.5, -29)
  line L19 (86.5, -29) -> (86.5, -27.2432)
  arc A18 (86.5, 22.3568) -> (86.5, 27.2432) centre (88.5, 24.8) ccw
  arc A19 (-86.5, 27.2432) -> (-86.5, 22.3568) centre (-88.5, 24.8) ccw
  line L20 (-86.5, 22.3568) -> (-86.5, -22.3568)
  line L21 (-86.5, -27.2432) -> (-86.5, -29)
  line L22 (86.5, -22.3568) -> (86.5, 22.3568)
  line L23 (86.5, 27.2432) -> (86.5, 29)
  dimension "d623" = 39.2
  dimension "d624" = 38.7
  dimension "d625" = 33.7
  dimension "d921" = 0
  dimension "d922" = 0
  dimension "d923" = 0
  dimension "d924" = 0
  constraint perpendicular L12 L15
  constraint parallel L10 L15
  constraint parallel L12 L13
  measures "d623" distance of L4.start L6.end
  measures "d624" distance of L13.start L12.end
  measures "d625" vertical distance of L10.end L12.end
extrude "Extrude1" [suppressed]
sketch "Sketch2" plane through (0, 45, 0) normal (0, 1, 0) x (-1, 0, 0)
  line L0 (-142.6498, -18.6989) -> (-103.4498, -18.6989)
  line L1 (-103.4498, -18.6989) -> (-103.4498, 15.5011)
  line L2 (-103.4498, 15.5011) -> (-142.6498, 15.5011)
  line L3 (-142.6498, 15.5011) -> (-142.6498, -18.6989)
extrude "Extrude2" [suppressed]
sketch "Sketch3" plane through (0, 49.8, 0) normal (0, 1, 0) x (-1, 0, 0)
  line L0 (-142.6498, 15.5011) -> (-142.6498, -18.6989)
  line L1 (-142.6498, -18.6989) -> (-103.4498, -18.6989)
  line L2 (-103.4498, -18.6989) -> (-103.4498, 15.5011)
  line L3 (-103.4498, 15.5011) -> (-142.6498, 15.5011)
  circle A0 centre (-123.0498, -1.5989) radius 14
  dimension "d616" = 28
  dimension "d617" = 17.1
  dimension "d618" = 34.2
  dimension "d619" = 39.2
  dimension "d620" = 19.6
  measures "d616" diameter of A0
  measures "d617" distance of L1 A0.centre
  measures "d618" distance of L1 L3
  measures "d619" distance of L0 L2
  measures "d620" distance of L2 A0.centre
extrude "Extrude3" [suppressed]
sketch "Sketch4" plane through (0, 49.8, 0) normal (0, 1, 0) x (-1, 0, 0)
  circle A0 centre (-123.0498, -1.5989) radius 14
  line L0 (-142.6498, 15.5011) -> (-142.6498, -18.6989)
  line L1 (-142.6498, -18.6989) -> (-103.4498, -18.6989)
  line L2 (-103.4498, -18.6989) -> (-103.4498, 15.5011)
  line L3 (-103.4498, 15.5011) -> (-142.6498, 15.5011)
  line L4 (-103.9498, 15.0011) -> (-142.1498, 15.0011)
  line L5 (-142.1498, 15.0011) -> (-142.1498, -18.1989)
  line L6 (-142.1498, -18.1989) -> (-103.9498, -18.1989)
  line L7 (-103.9498, -18.1989) -> (-103.9498, 15.0011)
  dimension "d627" = -0.5
extrude "Extrude4" [suppressed]
sketch "Sketch10" plane through (0, 37.0807, 0) normal (0, 1, 0) x (-1, 0, 0)
  circle A0 centre (80.75, -16) radius 2.1574
  circle A1 centre (80.75, 16.2) radius 2.1574
  circle A2 centre (-80.25, -16) radius 2.1574
  circle A3 centre (-80.25, 16.2) radius 2.1574
  line L0 (-81.25, -11) -> (-83.25, -11)
  line L1 (-83.25, -11) -> (-83.25, -19)
  line L2 (-83.25, -19) -> (-75.25, -19)
  line L3 (-75.25, -19) -> (-75.25, -17)
  line L4 (-75.25, -17) -> (-44.95, -17)
  line L5 (-44.95, -17) -> (-44.95, -19)
  line L6 (-44.95, -19) -> (-36.95, -19)
  line L7 (-36.95, -19) -> (-36.95, -17)
  line L8 (-36.95, -17) -> (-3.75, -17)
  line L9 (-3.75, -17) -> (-3.75, -19)
  line L10 (-3.75, -19) -> (4.25, -19)
  line L11 (4.25, -19) -> (4.25, -17)
  line L12 (4.25, -17) -> (37.45, -17)
  line L13 (37.45, -17) -> (37.45, -19)
  line L14 (37.45, -19) -> (45.45, -19)
  line L15 (45.45, -19) -> (45.45, -17)
  line L16 (45.45, -17) -> (75.75, -17)
  line L17 (75.75, -17) -> (75.75, -19)
  line L18 (75.75, -19) -> (83.75, -19)
  line L19 (83.75, -19) -> (83.75, -11)
  line L20 (83.75, -11) -> (81.75, -11)
  line L21 (81.75, -11) -> (81.75, 11.2)
  line L22 (81.75, 11.2) -> (83.75, 11.2)
  line L23 (83.75, 11.2) -> (83.75, 19.2)
  line L24 (83.75, 19.2) -> (75.75, 19.2)
  line L25 (75.75, 19.2) -> (75.75, 17.2)
  line L26 (75.75, 17.2) -> (45.45, 17.2)
  line L27 (45.45, 17.2) -> (45.45, 19.2)
  line L28 (45.45, 19.2) -> (37.45, 19.2)
  line L29 (37.45, 19.2) -> (37.45, 17.2)
  line L30 (37.45, 17.2) -> (4.25, 17.2)
  line L31 (4.25, 17.2) -> (4.25, 19.2)
  line L32 (4.25, 19.2) -> (-3.75, 19.2)
  line L33 (-3.75, 19.2) -> (-3.75, 17.2)
  line L34 (-3.75, 17.2) -> (-36.95, 17.2)
  line L35 (-36.95, 17.2) -> (-36.95, 19.2)
  line L36 (-36.95, 19.2) -> (-44.95, 19.2)
  line L37 (-44.95, 19.2) -> (-44.95, 17.2)
  line L38 (-44.95, 17.2) -> (-75.25, 17.2)
  line L39 (-75.25, 17.2) -> (-75.25, 19.2)
  line L40 (-75.25, 19.2) -> (-83.25, 19.2)
  line L41 (-83.25, 19.2) -> (-83.25, 11.2)
  line L42 (-83.25, 11.2) -> (-81.25, 11.2)
  line L43 (-81.25, 11.2) -> (-81.25, -11)
  line L44 (-0.75, -11) -> (-0.75, 11.2)
  line L45 (-0.75, 11.2) -> (1.25, 11.2)
  line L46 (1.25, 11.2) -> (1.25, -11)
  line L47 (1.25, -11) -> (-0.75, -11)
  line L48 (-41.95, -11) -> (-41.95, 11.2)
  line L49 (-41.95, 11.2) -> (-39.95, 11.2)
  line L50 (-39.95, 11.2) -> (-39.95, -11)
  line L51 (-39.95, -11) -> (-41.95, -11)
  circle A4 centre (-61.55, 13) radius 3.1
  circle A5 centre (-20.35, 13) radius 3.1
  circle A6 centre (36.25, 0.1) radius 3.1
  circle A7 centre (77.45, 0.1) radius 3.1
  circle A8 centre (62.05, -12.8) radius 3.1
  circle A9 centre (20.85, -12.8) radius 3.1
  circle A10 centre (-4.95, 0.1) radius 3.1
  circle A11 centre (-61.55, -12.8) radius 3.1
  circle A12 centre (-46.15, 0.1) radius 3.1
  circle A13 centre (-20.35, -12.8) radius 3.1
  circle A14 centre (20.85, 13) radius 3.1
  circle A15 centre (62.05, 13) radius 3.1
  circle A16 centre (46.65, 0.1) radius 3.1
  circle A17 centre (5.45, 0.1) radius 3.1
  circle A18 centre (-35.75, 0.1) radius 3.1
  circle A19 centre (-76.95, 0.1) radius 3.1
  line L52 (9.65, 8.8) -> (32.05, 8.8)
  line L53 (32.05, 8.8) -> (32.05, -8.6)
  line L54 (32.05, -8.6) -> (9.65, -8.6)
  line L55 (9.65, -8.6) -> (9.65, 8.8)
  line L56 (-31.55, 8.8) -> (-9.15, 8.8)
  line L57 (-9.15, 8.8) -> (-9.15, -8.6)
  line L58 (-9.15, -8.6) -> (-31.55, -8.6)
  line L59 (-31.55, -8.6) -> (-31.55, 8.8)
  line L60 (73.25, 8.8) -> (73.25, -8.6)
  line L61 (73.25, -8.6) -> (50.85, -8.6)
  line L62 (50.85, -8.6) -> (50.85, 8.8)
  line L63 (50.85, 8.8) -> (73.25, 8.8)
  line L64 (-72.75, 8.8) -> (-50.35, 8.8)
  line L65 (-50.35, 8.8) -> (-50.35, -8.6)
  line L66 (-50.35, -8.6) -> (-72.75, -8.6)
  line L67 (-72.75, -8.6) -> (-72.75, 8.8)
  line L68 (42.45, 11.2) -> (42.45, -11)
  line L69 (42.45, -11) -> (40.45, -11)
  line L70 (40.45, -11) -> (40.45, 11.2)
  line L71 (40.45, 11.2) -> (42.45, 11.2)
  circle A20 centre (62.05, 13) radius 3.1
  circle A21 centre (46.65, 0.1) radius 3.1
  circle A22 centre (62.05, -12.8) radius 3.1
  circle A23 centre (77.45, 0.1) radius 3.1
sketch "Sketch5" plane through (0, 24.0807, 0) normal (0, 1, 0) x (-1, 0, 0)
  circle A0 centre (80.5, -16.1) radius 2.1574
  circle A1 centre (80.5, 16.1) radius 2.1574
  circle A2 centre (-80.5, -16.1) radius 2.1574
  circle A3 centre (-80.5, 16.1) radius 2.1574
  line L0 (-81.5, -11.1) -> (-83.5, -11.1)
  line L1 (-83.5, -11.1) -> (-83.5, -19.1)
  line L2 (-83.5, -19.1) -> (-75.5, -19.1)
  line L3 (-75.5, -19.1) -> (-75.5, -17.1)
  line L4 (-75.5, -17.1) -> (-45.2, -17.1)
  line L5 (-45.2, -17.1) -> (-45.2, -19.1)
  line L6 (-45.2, -19.1) -> (-37.2, -19.1)
  line L7 (-37.2, -19.1) -> (-37.2, -17.1)
  line L8 (-37.2, -17.1) -> (-4, -17.1)
  line L9 (-4, -17.1) -> (-4, -19.1)
  line L10 (-4, -19.1) -> (4, -19.1)
  line L11 (4, -19.1) -> (4, -17.1)
  line L12 (4, -17.1) -> (37.2, -17.1)
  line L13 (37.2, -17.1) -> (37.2, -19.1)
  line L14 (37.2, -19.1) -> (45.2, -19.1)
  line L15 (45.2, -19.1) -> (45.2, -17.1)
  line L16 (45.2, -17.1) -> (75.5, -17.1)
  line L17 (75.5, -17.1) -> (75.5, -19.1)
  line L18 (75.5, -19.1) -> (83.5, -19.1)
  line L19 (83.5, -19.1) -> (83.5, -11.1)
  line L20 (83.5, -11.1) -> (81.5, -11.1)
  line L21 (81.5, -11.1) -> (81.5, 11.1)
  line L22 (81.5, 11.1) -> (83.5, 11.1)
  line L23 (83.5, 11.1) -> (83.5, 19.1)
  line L24 (83.5, 19.1) -> (75.5, 19.1)
  line L25 (75.5, 19.1) -> (75.5, 17.1)
  line L26 (75.5, 17.1) -> (45.2, 17.1)
  line L27 (45.2, 17.1) -> (45.2, 19.1)
  line L28 (45.2, 19.1) -> (37.2, 19.1)
  line L29 (37.2, 19.1) -> (37.2, 17.1)
  line L30 (37.2, 17.1) -> (4, 17.1)
  line L31 (4, 17.1) -> (4, 19.1)
  line L32 (4, 19.1) -> (-4, 19.1)
  line L33 (-4, 19.1) -> (-4, 17.1)
  line L34 (-4, 17.1) -> (-37.2, 17.1)
  line L35 (-37.2, 17.1) -> (-37.2, 19.1)
  line L36 (-37.2, 19.1) -> (-45.2, 19.1)
  line L37 (-45.2, 19.1) -> (-45.2, 17.1)
  line L38 (-45.2, 17.1) -> (-75.5, 17.1)
  line L39 (-75.5, 17.1) -> (-75.5, 19.1)
  line L40 (-75.5, 19.1) -> (-83.5, 19.1)
  line L41 (-83.5, 19.1) -> (-83.5, 11.1)
  line L42 (-83.5, 11.1) -> (-81.5, 11.1)
  line L43 (-81.5, 11.1) -> (-81.5, -11.1)
  line L44 (-1, -11.1) -> (-1, 11.1)
  line L45 (-1, 11.1) -> (1, 11.1)
  line L46 (1, 11.1) -> (1, -11.1)
  line L47 (1, -11.1) -> (-1, -11.1)
  line L48 (-42.2, -11.1) -> (-42.2, 11.1)
  line L49 (-42.2, 11.1) -> (-40.2, 11.1)
  line L50 (-40.2, 11.1) -> (-40.2, -11.1)
  line L51 (-40.2, -11.1) -> (-42.2, -11.1)
  circle A4 centre (-61.8, 12.9) radius 3.1
  circle A5 centre (-20.6, 12.9) radius 3.1
  circle A6 centre (36, 0) radius 3.1
  circle A7 centre (77.2, 0) radius 3.1
  circle A8 centre (61.8, -12.9) radius 3.1
  circle A9 centre (20.6, -12.9) radius 3.1
  circle A10 centre (-5.2, 0) radius 3.1
  circle A11 centre (-61.8, -12.9) radius 3.1
  circle A12 centre (-46.4, 0) radius 3.1
  circle A13 centre (-20.6, -12.9) radius 3.1
  circle A14 centre (20.6, 12.9) radius 3.1
  circle A15 centre (61.8, 12.9) radius 3.1
  circle A16 centre (46.4, 0) radius 3.1
  circle A17 centre (5.2, 0) radius 3.1
  circle A18 centre (-36, 0) radius 3.1
  circle A19 centre (-77.2, 0) radius 3.1
  line L52 (9.4, 8.7) -> (31.8, 8.7)
  line L53 (31.8, 8.7) -> (31.8, -8.7)
  line L54 (31.8, -8.7) -> (9.4, -8.7)
  line L55 (9.4, -8.7) -> (9.4, 8.7)
  line L56 (-31.8, 8.7) -> (-9.4, 8.7)
  line L57 (-9.4, 8.7) -> (-9.4, -8.7)
  line L58 (-9.4, -8.7) -> (-31.8, -8.7)
  line L59 (-31.8, -8.7) -> (-31.8, 8.7)
  line L60 (73, 8.7) -> (73, -8.7)
  line L61 (73, -8.7) -> (50.6, -8.7)
  line L62 (50.6, -8.7) -> (50.6, 8.7)
  line L63 (50.6, 8.7) -> (73, 8.7)
  line L64 (-73, 8.7) -> (-50.6, 8.7)
  line L65 (-50.6, 8.7) -> (-50.6, -8.7)
  line L66 (-50.6, -8.7) -> (-73, -8.7)
  line L67 (-73, -8.7) -> (-73, 8.7)
  line L68 (42.2, 11.1) -> (42.2, -11.1)
  line L69 (42.2, -11.1) -> (40.2, -11.1)
  line L70 (40.2, -11.1) -> (40.2, 11.1)
  line L71 (40.2, 11.1) -> (42.2, 11.1)
  circle A20 centre (20.6, 12.9) radius 3.1
  line L72 (-1, -11.1) -> (1, -11.1)
  line L73 (1, -11.1) -> (1, 11.1)
  line L74 (1, 11.1) -> (-1, 11.1)
  line L75 (-1, 11.1) -> (-1, -11.1)
  circle A21 centre (20.6, -12.9) radius 3.1
  line L76 (4, -19.1) -> (37.2, -19.1)
  line L77 (37.2, -19.1) -> (37.2, -17.1)
  line L78 (37.2, -17.1) -> (4, -17.1)
  line L79 (4, -17.1) -> (4, -19.1)
  line L80 (42.2, 11.1) -> (40.2, 11.1)
  line L81 (40.2, 11.1) -> (40.2, -11.1)
  line L82 (40.2, -11.1) -> (42.2, -11.1)
  line L83 (42.2, -11.1) -> (42.2, 11.1)
  line L84 (37.2, 19.1) -> (4, 19.1)
  line L85 (4, 19.1) -> (4, 17.1)
  line L86 (4, 17.1) -> (37.2, 17.1)
  line L87 (37.2, 17.1) -> (37.2, 19.1)
  line L88 (39.6, -16.8333) -> (1.6, -16.8333)
  line L89 (1.6, -16.8333) -> (1.6, 16.6667)
  line L90 (1.6, 16.6667) -> (39.6, 16.6667)
  line L91 (39.6, 16.6667) -> (39.6, -16.8333)
  line L92 (39.6, -16.8333) -> (1.6, 16.6667) construction
  line L93 (1.6, -16.8333) -> (39.6, 16.6667) construction
  point P0 (5.2, 0)
  point P1 (20.6, -12.9)
  point P2 (20.6, -0.0833)
  dimension "d849" = 38
  dimension "d850" = 33.5
  dimension "d933" = 0
  dimension "d934" = 0
  dimension "d935" = 0
  constraint perpendicular L88 L89
  constraint parallel L88 L90
  constraint parallel L89 L91
  constraint horizontal L88
  constraint coincident L92 P2
  constraint coincident L93 P2
  measures "d849" distance of L89.end L90.end
  measures "d850" distance of L88.end L89.end
extrude "Extrude5" add sketch "Sketch5" against normal blind 1.8 contours L52 L53 L54 L55 | L88 L89 L90 L91
sketch "Sketch7" plane through (0, 24.0807, 0) normal (0, 1, 0) x (-1, 0, 0)
  circle A0 centre (20.6, -12.9) radius 3.1
  circle A1 centre (20.6, 12.9) radius 3.1
  circle A2 centre (5.2, 0) radius 3.1
  circle A3 centre (36, 0) radius 3.1
  line L0 (39.6, 16.6667) -> (1.6, 16.6667)
  line L1 (1.6, 16.6667) -> (1.6, -16.8333)
  line L2 (1.6, -16.8333) -> (39.6, -16.8333)
  line L3 (39.6, -16.8333) -> (39.6, 16.6667)
  line L4 (39.6, -16.8333) -> (1.6, -16.8333)
  line L5 (1.6, -16.8333) -> (1.6, 16.6667)
  line L6 (1.6, 16.6667) -> (39.6, 16.6667)
  line L7 (39.6, 16.6667) -> (39.6, -16.8333)
  dimension "d859" = 38
  constraint horizontal L4
  constraint vertical L5
  constraint horizontal L6
  constraint vertical L7
  constraint coincident L0.end L1.start
  constraint coincident L2.end L3.start
  measures "d859" distance of L2.end L1.end
extrude "Extrude7" add sketch "Sketch7" along normal blind 1.2 contours A0 | A1 | A2 | A3 | L0 L1 L2 L3 L4 L5 L6 L7
sketch "Sketch8" plane through (0, 25.2807, 0) normal (0, 1, 0) x (-1, 0, 0)
  line L0 (39.6, 16.6667) -> (1.6, 16.6667)
  line L1 (1.6, 16.6667) -> (1.6, -16.8333)
  line L2 (1.6, -16.8333) -> (39.6, -16.8333)
  line L3 (39.6, -16.8333) -> (39.6, 16.6667)
  circle A0 centre (20.6, -0.0833) radius 14
  dimension "d862" = 19
  dimension "d863" = 16.75
  dimension "d864" = 28
  dimension "d865" = 38
  dimension "d866" = 33.5
  measures "d862" distance of L1 A0.centre
  measures "d863" distance of L0 A0.centre
  measures "d864" diameter of A0
  measures "d865" distance of L1.end L2.end
  measures "d866" distance of L0.start L2.end
extrude "Extrude8" add sketch "Sketch8" along normal blind 15 contours A0
sketch "Sketch9" plane through (-1.6, 0, 0) normal (1, 0, 0) x (0, 0, -1)
  line L0 (-16.6667, 25.2807) -> (-16.6667, 22.2807)
  line L1 (-16.6667, 22.2807) -> (16.8333, 22.2807)
  line L2 (16.8333, 22.2807) -> (16.8333, 25.2807)
  line L3 (16.8333, 25.2807) -> (-16.6667, 25.2807)
component "Component" placed x (1, 0, 0) y (0, 1, 0) z (0, 0, 1) at (0, 0, 0)
equation "d612 = magnetDepth"